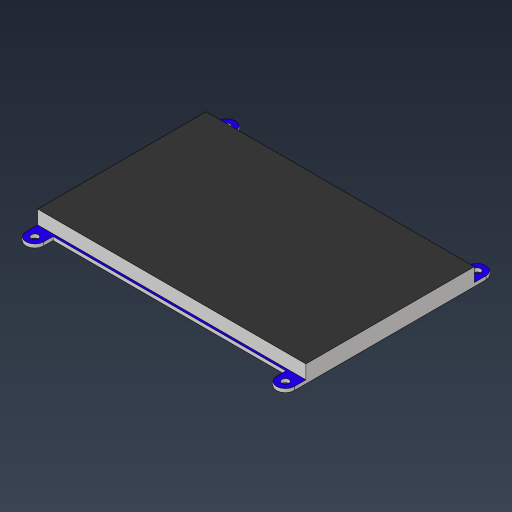
# Autodesk Inventor part: Display 5inch JRP5002
Saved by Autodesk Inventor 2023.1 (Build 271208000, 208)
## iProperties
Part Number: Display 5inch JRP5002
Material: Generisch
Document SubType Name: Modeling
Designer: rYan
Density: 1 g/cm^3
Appearance: Vorgabe
Author: rYan
Autodesk Inventor part; units mm, degrees
ref_plane "YZ Plane" through (0, 0, 0) normal (1, 0, 0) x (0, 1, 0)
sketch "Skizze1" plane through (0, 0, 0) normal (0, 0, 1) x (1, 0, 0)
  line L0 (-52.5, 39) -> (52.5, 39)
  line L1 (-52.5, -39) -> (52.5, -39)
  line L2 (52.5, -39) -> (52.5, -43.25)
  line L3 (-52.5, -39) -> (-52.5, -43.25)
  line L4 (-60.5, -43.25) -> (-60.5, 43.25)
  line L5 (-52.5, 39) -> (-52.5, 43.25)
  line L6 (52.5, 39) -> (52.5, 43.25)
  line L7 (60.5, 43.25) -> (60.5, -43.25)
  arc A0 (-52.5, 43.25) -> (-60.5, 43.25) centre (-56.5, 43.25) ccw
  arc A1 (60.5, 43.25) -> (52.5, 43.25) centre (56.5, 43.25) ccw
  arc A2 (52.5, -43.25) -> (60.5, -43.25) centre (56.5, -43.25) ccw
  arc A3 (-60.5, -43.25) -> (-52.5, -43.25) centre (-56.5, -43.25) ccw
  line L8 (0, 66.15) -> (0, -66.15) construction
  line L9 (-84.7, 0) -> (84.7, 0) construction
  circle A4 centre (-56.5, 43.25) radius 1.6
  circle A5 centre (56.5, 43.25) radius 1.6
  circle A6 centre (56.5, -43.25) radius 1.6
  circle A7 centre (-56.5, -43.25) radius 1.6
  point P0 (0, 0)
  dimension "d0" = 121
  dimension "d1" = 78
  dimension "d2" = 8
  dimension "d3" = 86.5
  dimension "d4" = 3.2
  constraints: 16 end point, 8 centre point, 8 point on circle, 8 tangent, 5 vertical, 4 coincident, 2 horizontal, 1 collinear, 1 perpendicular, 10 other
  measures "d0" distance between parallel lines of L7 L4
  measures "d1" distance between parallel lines of L1 L0
  measures "d2" distance between parallel lines of L7 L6
  measures "d3" distance of A2.centre A1.centre
  measures "d4" diameter of A4
extrude "Extrusion1" add sketch "Skizze1" along normal blind 1.6
sketch "Skizze2" plane through (0, 0, 1.6) normal (0, 0, 1) x (1, 0, 0)
  line L0 (-60.5, -38) -> (60.5, -38)
  line L1 (60.5, -38) -> (60.5, 38)
  line L2 (60.5, 38) -> (-60.5, 38)
  line L3 (-60.5, 38) -> (-60.5, -38)
  line L4 (-60.5, -38) -> (60.5, 38) construction
  line L5 (60.5, -38) -> (-60.5, 38) construction
  point P0 (0, 0)
  dimension "d7" = 76
  dimension "d8" = 121
  constraints: 12 end point, 2 midpoint, 2 parallel, 1 horizontal, 1 perpendicular
  measures "d7" distance of L2.end L0.start
  measures "d8" distance of L1.end L2.end
extrude "Extrusion2" add sketch "Skizze2" along normal blind 6.2
ref_plane "Arbeitsebene1" through (-52.5, 38.3, 0) normal (0, 1, 0) x (1, 0, 0)
sketch "Skizze3" plane through (-52.5, 38.3, 0) normal (0, 1, 0) x (1, 0, 0)
  line L0 (60.5, 2.5) -> (60.5, 1)
  line L1 (60.5, 1) -> (61.5, 0)
  line L2 (61.5, 0) -> (67, 0)
  line L3 (67, 0) -> (68, 1)
  line L4 (68, 1) -> (68, 2.5)
  line L5 (68, 2.5) -> (60.5, 2.5)
  line L6 (64.25, 2.5) -> (64.25, 0) construction
  line L7 (79.2, 2.5) -> (79.2, 1)
  line L8 (79.2, 1) -> (80.2, 0)
  line L9 (80.2, 0) -> (85.7, 0)
  line L10 (85.7, 0) -> (86.7, 1)
  line L11 (86.7, 1) -> (86.7, 2.5)
  line L12 (86.7, 2.5) -> (79.2, 2.5)
  line L13 (82.95, 2.5) -> (82.95, 0) construction
  line L14 (0, 0) -> (-8, 0) construction
  line L15 (105, 0) -> (0, 0) construction
  line L16 (113, 0) -> (105, 0) construction
  line L17 (105, 0) -> (113, 0) construction
  line L18 (0, 0) -> (105, 0) construction
  line L19 (-8, 0) -> (0, 0) construction
  line L20 (-2.4, 0) -> (-5.6, 0) construction
  line L21 (110.6, 0) -> (107.4, 0) construction
  line L22 (110.6, 0) -> (107.4, 0) construction
  line L23 (-2.4, 0) -> (-5.6, 0) construction
  line L24 (105, 0) -> (105, -1.6) construction
  line L25 (105, 0) -> (105, -1.6) construction
  point P0 (52.5, 0)
  dimension "d12" = 7.5
  dimension "d13" = 2.5
  dimension "d14" = 1.5
  dimension "d15" = 7.5
  dimension "d16" = 2.5
  dimension "d17" = 1.5
  dimension "d18" = 18.3
  dimension "d19" = 11.2
  constraints: 28 end point, 6 perpendicular, 4 midpoint, 4 vertical, 2 collinear, 2 parallel, 2 other
  measures "d12" distance of L4.end L0.start
  measures "d13" distance of L6.start L6.end
  measures "d14" distance of L0.start L0.end
  measures "d15" distance of L11.end L7.start
  measures "d16" distance of L13.start L13.end
  measures "d17" distance of L7.start L7.end
  measures "d18" distance between parallel lines of L11 L24
  measures "d19" distance between parallel lines of L4 L7
extrude "Extrusion3" add sketch "Skizze3" against normal blind 5.2
ref_plane "Arbeitsebene2" through (-52.5, 40.7, 0) normal (0, 1, 0) x (1, 0, 0)
sketch "Skizze4" plane through (-52.5, 40.7, 0) normal (0, 1, 0) x (1, 0, 0)
  line L0 (80.2, 0) -> (85.7, 0) projected
  line L1 (85.7, 0) -> (80.2, 0) projected
  line L2 (61.5, 0) -> (67, 0) projected
  line L3 (67, 0) -> (61.5, 0) projected
  line L4 (0, 0) -> (-8, 0) projected
  line L5 (105, 0) -> (0, 0) projected
  line L6 (113, 0) -> (105, 0) projected
  line L7 (105, 0) -> (113, 0) projected
  line L8 (0, 0) -> (105, 0) projected
  line L9 (-8, 0) -> (0, 0) projected
  line L10 (-2.4, 0) -> (-5.6, 0) projected
  line L11 (110.6, 0) -> (107.4, 0) projected
  line L12 (110.6, 0) -> (107.4, 0) projected
  line L13 (-2.4, 0) -> (-5.6, 0) projected
  line L14 (105, 0) -> (105, -1.6) projected
  line L15 (105, 0) -> (105, -1.6) projected
  line L16 (38.2, 6.4) -> (53.2, 6.4)
  line L17 (53.2, 6.4) -> (53.2, 2.4)
  line L18 (53.2, 2.4) -> (50.8, 0)
  line L19 (50.8, 0) -> (40.6, 0)
  line L20 (40.6, 0) -> (38.2, 2.4)
  line L21 (38.2, 2.4) -> (38.2, 6.4)
  line L22 (45.7, 6.4) -> (45.7, 0) construction
  point P0 (52.5, 0)
  point P1 (40.6, 0)
  point P2 (50.8, 0)
  dimension "d23" = 15
  dimension "d24" = 6.4
  dimension "d25" = 4
  dimension "d26" = 51.8
  constraints: 14 end point, 3 perpendicular, 2 midpoint, 1 collinear, 1 horizontal, 1 parallel, 1 vertical, 1 other
  measures "d23" distance of L16.start L16.end
  measures "d24" distance of L22.start L22.end
  measures "d25" distance of L20.end L16.start
  measures "d26" distance between parallel lines of L17 L14
extrude "Extrusion4" add sketch "Skizze4" against normal blind 12.2
sketch "Skizze5" plane through (-52.5, 39, 1.6) normal (0, 1, 0) x (1, 0, 0)
  line L0 (20.7, 6.6) -> (26.7, 6.6)
  line L1 (26.7, 6.6) -> (26.7, 1.6)
  line L2 (26.7, 1.6) -> (20.7, 1.6)
  line L3 (20.7, 1.6) -> (20.7, 6.6)
  line L4 (105, 1.6) -> (50.8, 1.6) projected
  line L5 (113, 1.6) -> (105, 1.6) projected
  line L6 (105, 1.6) -> (113, 1.6) projected
  line L7 (0, 1.6) -> (105, 1.6) projected
  line L8 (-8, 1.6) -> (0, 1.6) projected
  line L9 (0, 1.6) -> (-8, 1.6) projected
  line L10 (40.6, 1.6) -> (0, 1.6) projected
  line L11 (40.6, 1.6) -> (50.8, 1.6) projected
  line L12 (80.2, 1.6) -> (85.7, 1.6) projected
  line L13 (85.7, 1.6) -> (80.2, 1.6) projected
  line L14 (61.5, 1.6) -> (67, 1.6) projected
  line L15 (67, 1.6) -> (61.5, 1.6) projected
  line L16 (-2.4, 1.6) -> (-5.6, 1.6) projected
  line L17 (110.6, 1.6) -> (107.4, 1.6) projected
  line L18 (110.6, 1.6) -> (107.4, 1.6) projected
  line L19 (-2.4, 1.6) -> (-5.6, 1.6) projected
  line L20 (40.6, 1.6) -> (0, 1.6) projected
  line L21 (105, 1.6) -> (105, 0) projected
  point P0 (52.5, 1.6)
  dimension "d29" = 5
  dimension "d30" = 6
  dimension "d31" = 78.3
  constraints: 8 end point, 2 parallel, 1 collinear, 1 horizontal, 1 perpendicular
  measures "d29" distance of L0.end L1.end
  measures "d30" distance of L0.start L0.end
  measures "d31" distance between parallel lines of L1 L21
extrude "Extrusion5" add sketch "Skizze5" against normal blind 12.2
sketch "Skizze6" plane through (-52.5, 39, 1.6) normal (0, 1, 0) x (1, 0, 0)
  line L0 (26.7, 6.6) -> (20.7, 6.6) projected
  line L1 (20.7, 6.6) -> (20.7, 1.6) projected
  line L2 (26.7, 1.6) -> (26.7, 6.6) projected
  line L3 (20.7, 6.6) -> (26.7, 1.6) construction
  line L4 (26.7, 6.6) -> (20.7, 1.6) construction
  circle A0 centre (23.7, 4.1) radius 2.5
  circle A1 centre (23.7, 4.1) radius 1.5
  point P0 (52.5, 1.6)
  dimension "d34" = 3
  constraints: 4 end point, 2 centre point, 1 coincident, 1 midpoint, 1 tangent
  measures "d34" diameter of A1
extrude "Extrusion6" add sketch "Skizze6" along normal blind 1.8
sketch "Skizze7" plane through (0, 0, 0) normal (0, 0, -1) x (-1, 0, 0)
  line L0 (-42.3, 35.2) -> (-47.1, 35.2)
  line L1 (-47.1, 35.2) -> (-47.1, 38.8)
  line L2 (-42.3, 38.8) -> (-42.3, 35.2)
  line L3 (-46, 38.8) -> (-46, 40)
  line L4 (-46, 40) -> (-43.4, 40)
  line L5 (-43.4, 40) -> (-43.4, 38.8)
  line L6 (-47.1, 38.8) -> (-46, 38.8)
  line L7 (-43.4, 38.8) -> (-42.3, 38.8)
  line L8 (-44.7, 35.2) -> (-44.7, 40) construction
  line L9 (-52.5, 43.25) -> (-52.5, 39) construction
  line L10 (-52.5, 39) -> (1.7, 39) construction
  point P0 (0, 0)
  dimension "d37" = 2.6
  dimension "d38" = 1.2
  dimension "d39" = 3.6
  dimension "d40" = 4.8
  dimension "d41" = 5.4
  dimension "d42" = 1
  constraints: 18 end point, 4 parallel, 2 horizontal, 2 midpoint, 1 perpendicular, 3 other
  measures "d37" distance of L3.end L4.end
  measures "d38" distance of L3.start L3.end
  measures "d39" distance of L0.end L1.end
  measures "d40" distance of L0.start L0.end
  measures "d41" distance between parallel lines of L1 L9
  measures "d42" distance between parallel lines of L10 L4
extrude "Extrusion7" add sketch "Skizze7" along normal blind 1.8
